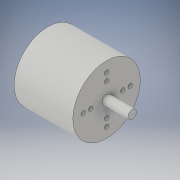
# Autodesk Inventor part: MotorModel
Saved by Autodesk Inventor 2018 (Build 220112000, 112)
## iProperties
Created: 2019-06-10
Part Number: MotorModel
Material: Generic
Document SubType Name: Modeling
Designer: anirudh
Density: 1 g/cm^3
Appearance: Default
Author: anirudh
Autodesk Inventor part; units mm, degrees
ref_plane "YZ Plane" through (0, 0, 0) normal (1, 0, 0) x (0, 1, 0)
ref_plane "XZ Plane" through (0, 0, 0) normal (0, 1, 0) x (-1, 0, 0)
ref_plane "XY Plane" through (0, 0, 0) normal (0, 0, 1) x (1, 0, 0)
sketch "Sketch1" plane through (0, 0, 0) normal (1, 0, 0) x (0, 1, 0)
  circle A0 centre (0, 0) radius 31.5
  dimension "d0" = 63
  constraints: 1 centre point, 1 coincident
  measures "d0" diameter of A0
extrude "Extrusion1" add sketch "Sketch1" along normal blind 75
sketch "Sketch2" plane through (75, 0, 0) normal (1, 0, 0) x (0, 0, -1)
  circle A0 centre (0, 0) radius 4
  dimension "d3" = 8
  constraints: 1 centre point, 1 coincident
  measures "d3" diameter of A0
extrude "Extrusion2" add sketch "Sketch2" along normal blind 24
sketch "Sketch3" plane through (75, 0, 0) normal (1, 0, 0) x (0, 0, -1)
  circle A0 centre (0, 15) radius 2
  circle A1 centre (0, 22) radius 2
  circle A2 centre (15, 0) radius 2
  circle A3 centre (22, 0) radius 2
  circle A4 centre (0, -15) radius 2
  circle A5 centre (0, -22) radius 2
  circle A6 centre (-15, 0) radius 2
  circle A7 centre (-22, 0) radius 2
  point P0 (0, 0)
  dimension "d8" = 4
  dimension "d9" = 4
  dimension "d10" = 4
  dimension "d11" = 4
  dimension "d12" = 4
  dimension "d13" = 4
  dimension "d14" = 4
  dimension "d15" = 4
  constraints: 8 centre point
  measures "d8" diameter of A0
  measures "d9" diameter of A1
  measures "d10" diameter of A2
  measures "d11" diameter of A3
  measures "d12" diameter of A4
  measures "d13" diameter of A5
  measures "d14" diameter of A6
  measures "d15" diameter of A7
extrude "Extrusion3" cut sketch "Sketch3" against normal blind 8
sketch "Sketch4" plane through (0, 0, 0) normal (-1, 0, 0) x (0, 0, 1)
  circle A0 centre (0, 0) radius 4 projected
  circle A1 centre (0, 0) radius 31.5
  constraints: 1 centre point, 1 coincident
extrude "Extrusion4" cut sketch "Sketch4" against normal blind 20 contours A0 | A1
sketch "Sketch5" plane through (75, 0, 0) normal (1, 0, 0) x (0, 0, -1)
  arc A0 (22.2739, -22.2739) -> (-22.2739, -22.2739) centre (0, 0) ccw
  arc A1 (17.3205, -10) -> (-17.3205, -10) centre (0, 0) ccw
  arc A2 (11.2583, -6.5) -> (-11.2583, -6.5) centre (0, 0) ccw
  arc A3 (14.7224, -8.5) -> (-14.7224, -8.5) centre (0, 0) ccw
  arc A4 (20.7846, -12) -> (-20.7846, -12) centre (0, 0) ccw
  line L0 (0, 0) -> (31.5, 0) construction
  arc A5 (-20.7846, -12) -> (-17.3205, -10) centre (-19.0526, -11) ccw
  arc A6 (-14.7224, -8.5) -> (-11.2583, -6.5) centre (-12.9904, -7.5) ccw
  arc A7 (11.2583, -6.5) -> (14.7224, -8.5) centre (12.9904, -7.5) ccw
  arc A8 (17.3205, -10) -> (20.7846, -12) centre (19.0526, -11) ccw
  line L1 (0, 0) -> (31.5, 0) construction
  line L2 (0, 0) -> (-2.8284, -2.8284)
  line L3 (-9.1924, -9.1924) -> (-22.2739, -22.2739)
  line L4 (9.1924, -9.1924) -> (22.2739, -22.2739)
  arc A9 (-9.1924, -9.1924) -> (9.1924, -9.1924) centre (0, 0) ccw
  arc A10 (11.2583, -6.5) -> (-11.2583, -6.5) centre (0, 0) ccw
  circle A11 centre (0, 0) radius 5
  dimension "d23" = 10
  constraints: 22 point on circle, 12 centre point, 10 end point, 7 coincident, 2 horizontal
  measures "d23" diameter of A11
body "Solid1"
